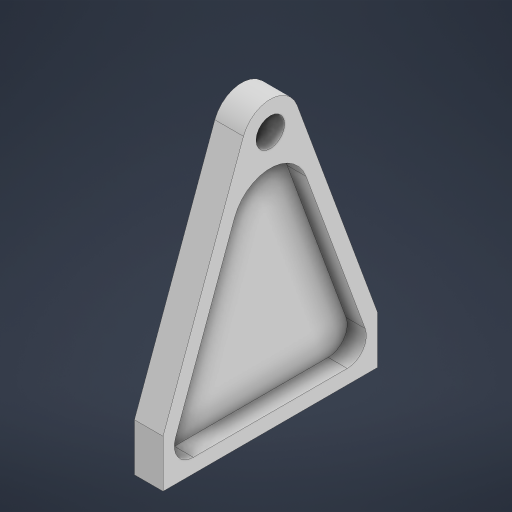
# Autodesk Inventor part: Bearing Short
Saved by Autodesk Inventor 2023.2 (Build 272271000, 271)
## iProperties
Created: 2023-01-17
Part Number: Bearing Short
Material: Generic
Document SubType Name: Modeling
Designer: iusti
Density: 1 g/cm^3
Appearance: Default
Author: iusti
Autodesk Inventor part; units mm, degrees
ref_plane "YZ Plane" through (0, 0, 0) normal (1, 0, 0) x (0, 1, 0)
ref_plane "XZ Plane" through (0, 0, 0) normal (0, 1, 0) x (-1, 0, 0)
ref_plane "XY Plane" through (0, 0, 0) normal (0, 0, 1) x (1, 0, 0)
sketch "Sketch1" plane through (0, 0, 0) normal (1, 0, 0) x (0, 1, 0)
  line L0 (0, 22.5) -> (0, -22.5)
  arc A0 (56.0629, -5.6342) -> (56.0629, 5.6342) centre (54, 0) ccw
  line L1 (0, 22.5) -> (10, 22.5)
  line L2 (0, -22.5) -> (10, -22.5)
  line L3 (10, -22.5) -> (56.0629, -5.6342)
  line L4 (10, 22.5) -> (56.0629, 5.6342)
  point P0 (0, 0)
  dimension "d1" = 6
  dimension "d2" = 10
  dimension "d3" = 54
  dimension "d4" = 45
  constraints: 10 end point, 2 horizontal, 2 midpoint, 2 point on circle, 2 tangent, 1 centre point, 1 horizontal alignment, 1 parallel, 1 vertical
  measures "d1" radius of A0
  measures "d2" distance of L0.start L1.end
  measures "d3" distance from line of L0 A0.centre
  measures "d4" distance between parallel lines of L2 L1
extrude "Extrusion1" add sketch "Sketch1" along normal blind 6
sketch "Sketch2" plane through (6, 0, 0) normal (1, 0, 0) x (0, 0, -1)
  line L0 (-22.5, 0) -> (22.5, 0) projected
  line L1 (22.5, 10) -> (5.6342, 56.0629) projected
  line L2 (-5.6342, 56.0629) -> (-22.5, 10) projected
  line L3 (-7.5123, 42.2083) -> (-19.9001, 8.3753)
  line L4 (-16.144, 3) -> (16.144, 3)
  line L5 (19.9001, 8.3753) -> (7.5123, 42.2083)
  arc A0 (7.5123, 42.2083) -> (-7.5123, 42.2083) centre (0, 39.4577) ccw
  arc A1 (-19.9001, 8.3753) -> (-16.144, 3) centre (-16.144, 7) ccw
  arc A2 (16.144, 3) -> (19.9001, 8.3753) centre (16.144, 7) ccw
  point P0 (0, 0)
  dimension "d8" = 4
  dimension "d9" = 8
  dimension "d10" = 3
  dimension "d11" = 3
  dimension "d12" = 3
  constraints: 6 end point, 6 point on circle, 6 tangent, 3 centre point, 2 parallel, 1 equal radius, 1 horizontal
  measures "d8" radius of A1
  measures "d9" radius of A0
  measures "d10" distance between parallel lines of L5 L1
  measures "d11" distance between parallel lines of L2 L3
  measures "d12" distance between parallel lines of L4 L0
extrude "Extrusion2" cut sketch "Sketch2" against normal blind 4
sketch "Sketch3" plane through (6, 0, 0) normal (1, 0, 0) x (0, 0, -1)
  arc A0 (5.6342, 56.0629) -> (-5.6342, 56.0629) centre (0, 54) ccw projected
  point P0 (0, 0)
  constraints: 1 coincident
hole "Hole1" at (6, 54, 0) direction (-1, 0, 0) diameter 6 end through all
body "Solid1"
